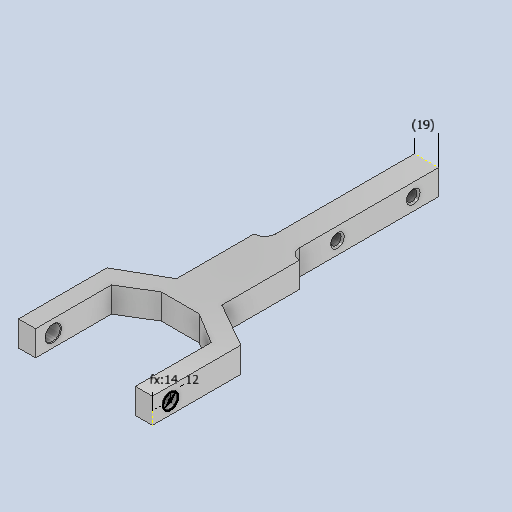
# Autodesk Inventor part: Adaptationhorizontalachse
Saved by Autodesk Inventor 2022 (Build 260153000, 153)
## iProperties
Created: 2022-02-28
Part Number: Adaptationhorizontalachse
Material: Aluminum 6061-AHC
Document SubType Name: Modeling
Designer: 123St
Density: 2.7 g/cm^3
Appearance: Aluminium - dunkel
Mass: 545.595 g
Surface Area: 397.771 cm^2
Volume: 202.072 cm^3
Fixation_dist1: -20,000 mm
Fixation_dist2: -60,000 mm
Gabel_FixierungPart_Width: 19,000 mm
Author: 123St
Autodesk Inventor part; units mm, degrees
ref_plane "YZ Plane" through (0, 0, 0) normal (1, 0, 0) x (0, 1, 0)
sketch "Skizze1" plane through (0, 0, 0) normal (0, 1, 0) x (-1, 0, 0)
  line L0 (53, 90) -> (53, 20)
  line L1 (53, 20) -> (18, 0)
  line L2 (18, 0) -> (-18, 0)
  line L3 (-18, 0) -> (-53, 20)
  line L4 (-53, 20) -> (-53, 90)
  line L5 (-53, 90) -> (-39.5, 90)
  line L6 (-39.5, 90) -> (-39.5, 30)
  line L7 (-39.5, 30) -> (-15, 15)
  line L8 (-15, 15) -> (15, 15)
  line L9 (15, 15) -> (39.5, 30)
  line L10 (39.5, 30) -> (39.5, 90)
  line L11 (39.5, 90) -> (53, 90)
  line L12 (0, -234) -> (0, 144) construction
  point P0 (0, 0)
  dimension "d0" = 79
  dimension "d1" = 13.5
  dimension "d2" = 13.5
  dimension "d3" = 90
  dimension "d5" = 60
  dimension "d6" = 15
  dimension "d7" = 60
  dimension "d8" = 70
  dimension "d9" = 70
  dimension "d12" = 15
  dimension "d13" = 15
  dimension "d14" = 18
  dimension "d15" = 18
  constraints: 24 end point, 4 perpendicular, 3 parallel, 1 equal length, 1 midpoint, 1 point on line, 1 vertical
  measures "d0" distance between parallel lines of L6 L10
  measures "d1" distance between parallel lines of L10 L0
  measures "d2" distance of L4.end L5.end
  measures "d3" distance between parallel lines of L11 L2
  measures "d5" distance of L9.end L10.end
  measures "d6" vertical distance of L9.end L8.end
  measures "d7" distance of L5.end L6.end
  measures "d8" distance of L0.start L0.end
  measures "d9" distance of L3.end L4.end
  measures "d12" distance from line of L8.end L12
  measures "d13" distance from line of L12 L7.end
  measures "d14" distance from line of L12 L1.end
  measures "d15" distance from line of L12 L2.end
extrude "Extrusion1" add sketch "Skizze1" along normal blind 20
sketch "Skizze2" plane through (18, 0, 0) normal (0, 0, -1) x (-1, 0, 0)
  line L0 (57.5, 20) -> (33, 20) construction
  line L1 (8.5, 0) -> (27.5, 0)
  line L2 (27.5, 0) -> (27.5, 20)
  line L3 (27.5, 20) -> (8.5, 20)
  line L4 (8.5, 20) -> (8.5, 0)
  line L5 (18, -4) -> (18, 24) construction
  line L6 (0, 0) -> (36, 0) construction
  point P0 (18, 0)
  point P1 (18, 0)
  point P2 (18, 20)
  dimension "d75" = 19
  constraints: 8 end point, 3 midpoint, 2 parallel, 2 point on line, 1 horizontal, 1 perpendicular
  measures "d75" distance between parallel lines of L2 L4
extrude "Extrusion2" add sketch "Skizze2" along normal blind 180
ref_plane "Arbeitsebene1" through (53.5, 2, 88) normal (1, 0, 0) x (0, 0, -1)
sketch "Skizze3" plane through (53, 0, 90) normal (1, 0, 0) x (0, 0, -1)
  line L0 (0, 10) -> (14, 10) construction
  line L1 (0, 0) -> (0, 20) construction
  circle A0 centre (14, 10) radius 6
  dimension "d44" = 14
  dimension "d87" = 12
  constraints: 2 end point, 1 centre point, 1 coincident, 1 horizontal, 1 midpoint
  measures "d44" distance of L0.start L0.end
  measures "d87" diameter of A0
extrude "Extrusion3" cut sketch "Skizze3" against normal through all
ref_plane "Arbeitsebene5" through (18, 0, -160) normal (0, 0, -1) x (-1, 0, 0)
ref_plane "Arbeitsebene6" through (18, 0, -100) normal (0, 0, -1) x (-1, 0, 0)
ref_plane "Arbeitsebene7" through (18, 0, -130) normal (0, 0, -1) x (-1, 0, 0)
sketch "Skizze13" plane through (9.5, 0, 0) normal (1, 0, 0) x (0, 0, -1)
  line L0 (160, 24) -> (160, -4) construction
  line L1 (100, 24) -> (100, -4) construction
  line L2 (180, 0) -> (180, 20) construction
  line L3 (180, 10) -> (100, 10) construction
  point P0 (0, 0)
  point P1 (160, 10)
  constraints: 3 midpoint, 2 end point, 1 coincident, 1 perpendicular, 1 point on line
hole "Bohrung2" at (9.5, 10, -100) at (9.5, 10, -160) direction (-1, 0, 0) diameter 8.376 end through all thread size "M10x1.5" class "6H" standard "ISO Metric profile"
sketch "Skizze11" plane through (0, 20, 0) normal (0, 1, 0) x (1, 0, 0)
  line L0 (9.5, 0) -> (18, 0)
  line L1 (18, 0) -> (18, 61.5)
  line L2 (9.5, 70) -> (9.5, 0)
  line L3 (-9.5, 0) -> (-9.5, 180) projected
  line L4 (-9.5, 0) -> (-18, 0)
  line L5 (-18, 0) -> (-18, 61.5)
  line L6 (-9.5, 70) -> (-9.5, 0)
  arc A0 (9.5, 70) -> (18, 61.5) centre (18, 70) ccw
  arc A1 (-18, 61.5) -> (-9.5, 70) centre (-18, 70) ccw
  point P0 (0, 0)
  point P1 (-9.5, 70)
  dimension "d80" = 70
  dimension "d81" = 70
  constraints: 12 end point, 4 point on circle, 2 centre point, 2 horizontal, 2 line through centre, 2 parallel, 2 perpendicular, 2 tangent
  measures "d80" distance from line of L0 L2.start
  measures "d81" distance from line of L4 L6.start
extrude "Extrusion7" add sketch "Skizze11" against normal up to surface (20 mm away)
sketch "Skizze12" plane through (18, 0, -180) normal (0, 0, -1) x (-1, 0, 0)
  line L0 (27.5, 20) -> (8.5, 20) construction
  point P0 (18, 0)
  dimension "Gabel_FixierungPart_Width" = 19
  measures "Gabel_FixierungPart_Width" distance of L0.start L0.end
chamfer "Fase1" distance 1.25 angle 45 4 edges at (9.5, 10, -155.812) (9.5, 10, -95.812) (-9.5, 10, -155.812) (-9.5, 10, -95.812)
chamfer "Fase2" distance 0.5 angle 45 4 edges at (53, 10, 82) (39.5, 10, 82) (-53, 10, 82) (-39.5, 10, 82)
equation "\"d1\" = d2"
equation "\"d75\" = ParallelMecha_Contact_Dist - 2 * Gabel_FixationShaft_Contact_Thickness"
equation "\"d81\" = d80"
equation "\"Fixation_dist2\" = -Total_Bearing_Hole_Dist"
equation "\"ParallelMecha_Contact_Dist\" = 26"
equation "\"Gabel_FixationShaft_Contact_Thickness\" = 3.5"
equation "\"Total_Bearing_Hole_Dist\" = 60"
